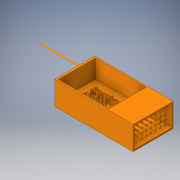
# Autodesk Inventor part: receiver
Saved by Autodesk Inventor 2016 (Build 200138000, 138)
## iProperties
Created: 2015-05-26
Part Number: receiver
Material: Generic
Document SubType Name: Modeling
Designer: Admin
Density: 1 g/cm^3
Appearance: Diamond plate 2 - Dark Gray
Mass: 3.8719 g
Surface Area: 64.7875 cm^2
Volume: 3.8719 cm^3
Author: Admin
Autodesk Inventor part; units mm, degrees
ref_plane "YZ Plane" through (0, 0, 0) normal (1, 0, 0) x (0, 1, 0)
ref_plane "XZ Plane" through (0, 0, 0) normal (0, 1, 0) x (-1, 0, 0)
ref_plane "XY Plane" through (0, 0, 0) normal (0, 0, 1) x (1, 0, 0)
sketch "Sketch1" plane through (0, 0, 0) normal (0, 1, 0) x (-1, 0, 0)
  line L0 (0, 0) -> (43, 0)
  line L1 (43, 0) -> (43, -22)
  line L2 (43, -22) -> (0, -22)
  line L3 (0, -22) -> (0, 0)
  dimension "d0" = 43
  dimension "d1" = 22
  constraints: 8 end point, 2 parallel, 1 horizontal, 1 perpendicular
  measures "d0" distance of L1.end L2.end
  measures "d1" distance of L0.end L1.end
extrude "Extrusion1" add sketch "Sketch1" along normal blind 13
sketch "Sketch2" plane through (0, 0, 0) normal (1, 0, 0) x (0, 0, -1)
  line L0 (0.8065, 0.8735) -> (21.1935, 0.8735)
  line L1 (21.1935, 0.8735) -> (21.1935, 12.1265)
  line L2 (21.1935, 12.1265) -> (0.8065, 12.1265)
  line L3 (0.8065, 12.1265) -> (0.8065, 0.8735)
  line L4 (0.8065, 0.8735) -> (21.1935, 12.1265) construction
  line L5 (21.1935, 0.8735) -> (0.8065, 12.1265) construction
  point P0 (0, 0)
  point P1 (11, 6.5)
  constraints: 12 end point, 2 midpoint, 2 parallel, 1 horizontal, 1 perpendicular
extrude "Extrusion2" cut sketch "Sketch2" against normal blind 13
sketch "Sketch3" plane through (-13, 0, 0) normal (1, 0, 0) x (0, 0, -1)
  circle A0 centre (4.65, 6.5) radius 0.4445
  circle A1 centre (4.65, 9.04) radius 0.4445
  circle A2 centre (4.65, 3.96) radius 0.4445
  line L0 (0.8065, 0.8735) -> (0.8065, 12.1265) projected
  line L1 (21.1935, 12.1265) -> (21.1935, 0.8735) projected
  circle A3 centre (9.73, 6.5) radius 0.4445
  circle A4 centre (9.73, 9.04) radius 0.4445
  circle A5 centre (9.73, 3.96) radius 0.4445
  circle A6 centre (7.19, 9.04) radius 0.4445
  circle A7 centre (7.19, 6.5) radius 0.4445
  circle A8 centre (7.19, 3.96) radius 0.4445
  circle A9 centre (17.35, 6.5) radius 0.4445
  circle A10 centre (17.35, 9.04) radius 0.4445
  circle A11 centre (17.35, 3.96) radius 0.4445
  circle A12 centre (12.27, 9.04) radius 0.4445
  circle A13 centre (12.27, 6.5) radius 0.4445
  circle A14 centre (12.27, 3.96) radius 0.4445
  circle A15 centre (14.81, 9.04) radius 0.4445
  circle A16 centre (14.81, 6.5) radius 0.4445
  circle A17 centre (14.81, 3.96) radius 0.4445
  point P0 (0, 0)
  constraints: 18 centre point
extrude "Extrusion3" add sketch "Sketch3" along normal blind 13
sketch "Sketch4" plane through (0, 13, 0) normal (0, 1, 0) x (1, 0, 0)
  line L0 (-41.9002, 0.8065) -> (-14.0998, 0.8065)
  line L1 (-14.0998, 0.8065) -> (-14.0998, 21.1935)
  line L2 (-14.0998, 21.1935) -> (-41.9002, 21.1935)
  line L3 (-41.9002, 21.1935) -> (-41.9002, 0.8065)
  line L4 (-41.9002, 0.8065) -> (-14.0998, 21.1935) construction
  line L5 (-14.0998, 0.8065) -> (-41.9002, 21.1935) construction
  point P0 (-13, 21.1935)
  point P1 (-13, 0.8065)
  point P2 (-28, 11)
  constraints: 12 end point, 2 midpoint, 2 parallel, 1 horizontal, 1 perpendicular
extrude "Extrusion4" cut sketch "Sketch4" against normal blind 10
sketch "Sketch5" plane through (0, 3, 0) normal (0, 1, 0) x (1, 0, 0)
  line L0 (-36.0677, 15.3871) -> (-11.819, 15.3871) construction
  line L1 (-11.819, 15.3871) -> (-11.819, -1.6232) construction
  line L2 (-11.819, -1.6232) -> (-36.0677, -1.6232) construction
  line L3 (-36.0677, -1.6232) -> (-36.0677, 15.3871) construction
  line L4 (-33.4001, 12.3193) -> (-33.9262, 12.3193)
  line L5 (-33.9262, 12.3193) -> (-34.8895, 13.5321)
  line L6 (-34.8895, 13.5321) -> (-35.3538, 13.5321)
  line L7 (-35.3538, 13.5321) -> (-35.3538, 12.3193)
  line L8 (-35.3538, 12.3193) -> (-35.7589, 12.3193)
  line L9 (-35.7589, 12.3193) -> (-35.7589, 15.3673)
  line L10 (-35.7589, 15.3673) -> (-34.9735, 15.3673)
  spline S0 degree 2 poles (-34.9735, 15.3673) (-34.7116, 15.3673) (-34.3584, 15.3105) (-34.1979, 15.2067) knots 0 0 0 1 2 2 2
  spline S1 degree 2 poles (-34.1979, 15.2067) (-34.0373, 15.103) (-33.8521, 14.7794) (-33.8521, 14.5398) knots 0 0 0 1 2 2 2
  spline S2 degree 2 poles (-33.8521, 14.5398) (-33.8521, 14.2064) (-34.1929, 13.7544) (-34.4844, 13.6457) knots 0 0 0 1 2 2 2
  line L11 (-34.4844, 13.6457) -> (-33.4001, 12.3193)
  spline S3 degree 2 poles (-34.2744, 14.5077) (-34.2744, 14.6411) (-34.3683, 14.8461) (-34.4671, 14.9128) knots 0 0 0 1 2 2 2
  spline S4 degree 2 poles (-34.4671, 14.9128) (-34.5536, 14.9696) (-34.7833, 15.0166) (-34.9512, 15.0166) knots 0 0 0 1 2 2 2
  line L12 (-34.9512, 15.0166) -> (-35.3538, 15.0166)
  line L13 (-35.3538, 15.0166) -> (-35.3538, 13.8705)
  line L14 (-35.3538, 13.8705) -> (-34.9982, 13.8705)
  spline S5 degree 2 poles (-34.9982, 13.8705) (-34.8228, 13.8705) (-34.5437, 13.9322) (-34.4473, 14.0286) knots 0 0 0 1 2 2 2
  spline S6 degree 2 poles (-34.4473, 14.0286) (-34.3584, 14.1125) (-34.2744, 14.3497) (-34.2744, 14.5077) knots 0 0 0 1 2 2 2
  spline S7 degree 2 poles (-32.1947, 12.2674) (-32.743, 12.2674) (-33.3457, 12.8825) (-33.3457, 13.4506) knots 0 0 0 1 2 2 2
  spline S8 degree 2 poles (-33.3457, 13.4506) (-33.3457, 14.0088) (-32.7603, 14.6708) (-32.2886, 14.6708) knots 0 0 0 1 2 2 2
  spline S9 degree 2 poles (-32.2886, 14.6708) (-32.0761, 14.6708) (-31.7476, 14.5473) (-31.6266, 14.4163) knots 0 0 0 1 2 2 2
  spline S10 degree 2 poles (-31.6266, 14.4163) (-31.5031, 14.2854) (-31.3722, 13.9075) (-31.3722, 13.6333) knots 0 0 0 1 2 2 2
  line L15 (-31.3722, 13.6333) -> (-31.3722, 13.4234)
  line L16 (-31.3722, 13.4234) -> (-32.9555, 13.4234)
  spline S11 degree 2 poles (-32.9555, 13.4234) (-32.9555, 13.0257) (-32.5553, 12.6034) (-32.1996, 12.6034) knots 0 0 0 1 2 2 2
  spline S12 degree 2 poles (-32.1996, 12.6034) (-32.0737, 12.6034) (-31.8291, 12.6602) (-31.7303, 12.7046) knots 0 0 0 1 2 2 2
  spline S13 degree 2 poles (-31.7303, 12.7046) (-31.6266, 12.754) (-31.4833, 12.8405) (-31.4364, 12.88) knots 0 0 0 1 2 2 2
  line L17 (-31.4364, 12.88) -> (-31.4142, 12.88)
  line L18 (-31.4142, 12.88) -> (-31.4142, 12.4601)
  spline S14 degree 2 poles (-31.4142, 12.4601) (-31.4809, 12.4329) (-31.6834, 12.3539) (-31.7624, 12.3317) knots 0 0 0 1 2 2 2
  spline S15 degree 2 poles (-31.7624, 12.3317) (-31.8736, 12.2995) (-32.0564, 12.2674) (-32.1947, 12.2674) knots 0 0 0 1 2 2 2
  spline S16 degree 2 poles (-31.7476, 13.7173) (-31.7526, 13.8729) (-31.8168, 14.1002) (-31.8785, 14.1768) knots 0 0 0 1 2 2 2
  spline S17 degree 2 poles (-31.8785, 14.1768) (-31.9452, 14.2632) (-32.1552, 14.3546) (-32.3108, 14.3546) knots 0 0 0 1 2 2 2
  spline S18 degree 2 poles (-32.3108, 14.3546) (-32.4639, 14.3546) (-32.6788, 14.2632) (-32.7677, 14.1743) knots 0 0 0 1 2 2 2
  spline S19 degree 2 poles (-32.7677, 14.1743) (-32.8542, 14.0829) (-32.9431, 13.8631) (-32.9555, 13.7173) knots 0 0 0 1 2 2 2
  line L19 (-32.9555, 13.7173) -> (-31.7476, 13.7173)
  spline S20 degree 2 poles (-30.0729, 12.2674) (-30.3101, 12.2674) (-30.7028, 12.4132) (-30.8436, 12.5614) knots 0 0 0 1 2 2 2
  spline S21 degree 2 poles (-30.8436, 12.5614) (-30.9844, 12.7071) (-31.14, 13.1566) (-31.14, 13.458) knots 0 0 0 1 2 2 2
  spline S22 degree 2 poles (-31.14, 13.458) (-31.14, 13.7593) (-30.9794, 14.199) (-30.8436, 14.3472) knots 0 0 0 1 2 2 2
  spline S23 degree 2 poles (-30.8436, 14.3472) (-30.7077, 14.4979) (-30.3051, 14.6584) (-30.0729, 14.6584) knots 0 0 0 1 2 2 2
  spline S24 degree 2 poles (-30.0729, 14.6584) (-29.8852, 14.6584) (-29.5345, 14.5522) (-29.3986, 14.483) knots 0 0 0 1 2 2 2
  line L20 (-29.3986, 14.483) -> (-29.3986, 14.0508)
  line L21 (-29.3986, 14.0508) -> (-29.4209, 14.0508)
  spline S25 degree 2 poles (-29.4209, 14.0508) (-29.4629, 14.0854) (-29.5913, 14.1743) (-29.6827, 14.2212) knots 0 0 0 1 2 2 2
  spline S26 degree 2 poles (-29.6827, 14.2212) (-29.7642, 14.2607) (-29.9816, 14.3225) (-30.0804, 14.3225) knots 0 0 0 1 2 2 2
  spline S27 degree 2 poles (-30.0804, 14.3225) (-30.3792, 14.3225) (-30.7423, 13.8705) (-30.7423, 13.458) knots 0 0 0 1 2 2 2
  spline S28 degree 2 poles (-30.7423, 13.458) (-30.7423, 13.0554) (-30.3916, 12.6034) (-30.0804, 12.6034) knots 0 0 0 1 2 2 2
  spline S29 degree 2 poles (-30.0804, 12.6034) (-29.8926, 12.6034) (-29.5518, 12.759) (-29.4209, 12.88) knots 0 0 0 1 2 2 2
  line L22 (-29.4209, 12.88) -> (-29.3986, 12.88)
  line L23 (-29.3986, 12.88) -> (-29.3986, 12.4477)
  spline S30 degree 2 poles (-29.3986, 12.4477) (-29.4554, 12.4206) (-29.6283, 12.344) (-29.6975, 12.3267) knots 0 0 0 1 2 2 2
  spline S31 degree 2 poles (-29.6975, 12.3267) (-29.7963, 12.2971) (-29.9519, 12.2674) (-30.0729, 12.2674) knots 0 0 0 1 2 2 2
  spline S32 degree 2 poles (-28.0549, 12.2674) (-28.6033, 12.2674) (-29.206, 12.8825) (-29.206, 13.4506) knots 0 0 0 1 2 2 2
  spline S33 degree 2 poles (-29.206, 13.4506) (-29.206, 14.0088) (-28.6206, 14.6708) (-28.1488, 14.6708) knots 0 0 0 1 2 2 2
  spline S34 degree 2 poles (-28.1488, 14.6708) (-27.9364, 14.6708) (-27.6079, 14.5473) (-27.4868, 14.4163) knots 0 0 0 1 2 2 2
  spline S35 degree 2 poles (-27.4868, 14.4163) (-27.3633, 14.2854) (-27.2324, 13.9075) (-27.2324, 13.6333) knots 0 0 0 1 2 2 2
  line L24 (-27.2324, 13.6333) -> (-27.2324, 13.4234)
  line L25 (-27.2324, 13.4234) -> (-28.8157, 13.4234)
  spline S36 degree 2 poles (-28.8157, 13.4234) (-28.8157, 13.0257) (-28.4156, 12.6034) (-28.0599, 12.6034) knots 0 0 0 1 2 2 2
  spline S37 degree 2 poles (-28.0599, 12.6034) (-27.9339, 12.6034) (-27.6894, 12.6602) (-27.5906, 12.7046) knots 0 0 0 1 2 2 2
  spline S38 degree 2 poles (-27.5906, 12.7046) (-27.4868, 12.754) (-27.3436, 12.8405) (-27.2967, 12.88) knots 0 0 0 1 2 2 2
  line L26 (-27.2967, 12.88) -> (-27.2744, 12.88)
  line L27 (-27.2744, 12.88) -> (-27.2744, 12.4601)
  spline S39 degree 2 poles (-27.2744, 12.4601) (-27.3411, 12.4329) (-27.5437, 12.3539) (-27.6227, 12.3317) knots 0 0 0 1 2 2 2
  spline S40 degree 2 poles (-27.6227, 12.3317) (-27.7338, 12.2995) (-27.9166, 12.2674) (-28.0549, 12.2674) knots 0 0 0 1 2 2 2
  spline S41 degree 2 poles (-27.6079, 13.7173) (-27.6128, 13.8729) (-27.677, 14.1002) (-27.7388, 14.1768) knots 0 0 0 1 2 2 2
  spline S42 degree 2 poles (-27.7388, 14.1768) (-27.8055, 14.2632) (-28.0154, 14.3546) (-28.171, 14.3546) knots 0 0 0 1 2 2 2
  spline S43 degree 2 poles (-28.171, 14.3546) (-28.3242, 14.3546) (-28.5391, 14.2632) (-28.628, 14.1743) knots 0 0 0 1 2 2 2
  spline S44 degree 2 poles (-28.628, 14.1743) (-28.7144, 14.0829) (-28.8034, 13.8631) (-28.8157, 13.7173) knots 0 0 0 1 2 2 2
  line L28 (-28.8157, 13.7173) -> (-27.6079, 13.7173)
  line L29 (-26.4494, 12.3193) -> (-26.8348, 12.3193)
  line L30 (-26.8348, 12.3193) -> (-26.8348, 14.6065)
  line L31 (-26.8348, 14.6065) -> (-26.4494, 14.6065)
  line L32 (-26.4494, 14.6065) -> (-26.4494, 12.3193)
  line L33 (-26.4223, 14.9869) -> (-26.8595, 14.9869)
  line L34 (-26.8595, 14.9869) -> (-26.8595, 15.3871)
  line L35 (-26.8595, 15.3871) -> (-26.4223, 15.3871)
  line L36 (-26.4223, 15.3871) -> (-26.4223, 14.9869)
  line L37 (-24.0881, 14.6065) -> (-24.9501, 12.3193)
  line L38 (-24.9501, 12.3193) -> (-25.2959, 12.3193)
  line L39 (-25.2959, 12.3193) -> (-26.1506, 14.6065)
  line L40 (-26.1506, 14.6065) -> (-25.7331, 14.6065)
  line L41 (-25.7331, 14.6065) -> (-25.1082, 12.8454)
  line L42 (-25.1082, 12.8454) -> (-24.4882, 14.6065)
  line L43 (-24.4882, 14.6065) -> (-24.0881, 14.6065)
  spline S45 degree 2 poles (-22.8037, 12.2674) (-23.352, 12.2674) (-23.9547, 12.8825) (-23.9547, 13.4506) knots 0 0 0 1 2 2 2
  spline S46 degree 2 poles (-23.9547, 13.4506) (-23.9547, 14.0088) (-23.3693, 14.6708) (-22.8976, 14.6708) knots 0 0 0 1 2 2 2
  spline S47 degree 2 poles (-22.8976, 14.6708) (-22.6851, 14.6708) (-22.3566, 14.5473) (-22.2356, 14.4163) knots 0 0 0 1 2 2 2
  spline S48 degree 2 poles (-22.2356, 14.4163) (-22.1121, 14.2854) (-21.9812, 13.9075) (-21.9812, 13.6333) knots 0 0 0 1 2 2 2
  line L44 (-21.9812, 13.6333) -> (-21.9812, 13.4234)
  line L45 (-21.9812, 13.4234) -> (-23.5645, 13.4234)
  spline S49 degree 2 poles (-23.5645, 13.4234) (-23.5645, 13.0257) (-23.1643, 12.6034) (-22.8086, 12.6034) knots 0 0 0 1 2 2 2
  spline S50 degree 2 poles (-22.8086, 12.6034) (-22.6827, 12.6034) (-22.4381, 12.6602) (-22.3393, 12.7046) knots 0 0 0 1 2 2 2
  spline S51 degree 2 poles (-22.3393, 12.7046) (-22.2356, 12.754) (-22.0923, 12.8405) (-22.0454, 12.88) knots 0 0 0 1 2 2 2
  line L46 (-22.0454, 12.88) -> (-22.0232, 12.88)
  line L47 (-22.0232, 12.88) -> (-22.0232, 12.4601)
  spline S52 degree 2 poles (-22.0232, 12.4601) (-22.0899, 12.4329) (-22.2924, 12.3539) (-22.3714, 12.3317) knots 0 0 0 1 2 2 2
  spline S53 degree 2 poles (-22.3714, 12.3317) (-22.4826, 12.2995) (-22.6654, 12.2674) (-22.8037, 12.2674) knots 0 0 0 1 2 2 2
  spline S54 degree 2 poles (-22.3566, 13.7173) (-22.3616, 13.8729) (-22.4258, 14.1002) (-22.4875, 14.1768) knots 0 0 0 1 2 2 2
  spline S55 degree 2 poles (-22.4875, 14.1768) (-22.5542, 14.2632) (-22.7642, 14.3546) (-22.9198, 14.3546) knots 0 0 0 1 2 2 2
  spline S56 degree 2 poles (-22.9198, 14.3546) (-23.0729, 14.3546) (-23.2878, 14.2632) (-23.3767, 14.1743) knots 0 0 0 1 2 2 2
  spline S57 degree 2 poles (-23.3767, 14.1743) (-23.4632, 14.0829) (-23.5521, 13.8631) (-23.5645, 13.7173) knots 0 0 0 1 2 2 2
  line L48 (-23.5645, 13.7173) -> (-22.3566, 13.7173)
  line L49 (-20.3781, 14.194) -> (-20.3979, 14.194)
  spline S58 degree 2 poles (-20.3979, 14.194) (-20.4424, 14.2064) (-20.5387, 14.2113) (-20.6054, 14.2113) knots 0 0 0 1 2 2 2
  spline S59 degree 2 poles (-20.6054, 14.2113) (-20.761, 14.2113) (-21.0673, 14.0755) (-21.2056, 13.9421) knots 0 0 0 1 2 2 2
  line L50 (-21.2056, 13.9421) -> (-21.2056, 12.3193)
  line L51 (-21.2056, 12.3193) -> (-21.5909, 12.3193)
  line L52 (-21.5909, 12.3193) -> (-21.5909, 14.6065)
  line L53 (-21.5909, 14.6065) -> (-21.2056, 14.6065)
  line L54 (-21.2056, 14.6065) -> (-21.2056, 14.2657)
  spline S60 degree 2 poles (-21.2056, 14.2657) (-20.9956, 14.4534) (-20.6819, 14.6065) (-20.5337, 14.6065) knots 0 0 0 1 2 2 2
  spline S61 degree 2 poles (-20.5337, 14.6065) (-20.4745, 14.6065) (-20.4152, 14.6016) (-20.3781, 14.5942) knots 0 0 0 1 2 2 2
  line L55 (-20.3781, 14.5942) -> (-20.3781, 14.194)
  spline S62 degree 2 poles (-34.5684, 7.2465) (-34.8648, 7.2465) (-35.3662, 7.4466) (-35.549, 7.6467) knots 0 0 0 1 2 2 2
  spline S63 degree 2 poles (-35.549, 7.6467) (-35.7318, 7.8443) (-35.9318, 8.4371) (-35.9318, 8.8224) knots 0 0 0 1 2 2 2
  spline S64 degree 2 poles (-35.9318, 8.8224) (-35.9318, 9.2052) (-35.7367, 9.7733) (-35.5514, 9.9833) knots 0 0 0 1 2 2 2
  spline S65 degree 2 poles (-35.5514, 9.9833) (-35.3687, 10.1883) (-34.8697, 10.4032) (-34.561, 10.4032) knots 0 0 0 1 2 2 2
  spline S66 degree 2 poles (-34.561, 10.4032) (-34.4078, 10.4032) (-34.1386, 10.3587) (-34.025, 10.3241) knots 0 0 0 1 2 2 2
  spline S67 degree 2 poles (-34.025, 10.3241) (-33.9262, 10.292) (-33.7212, 10.2006) (-33.6199, 10.1463) knots 0 0 0 1 2 2 2
  line L56 (-33.6199, 10.1463) -> (-33.6199, 9.6572)
  line L57 (-33.6199, 9.6572) -> (-33.652, 9.6572)
  spline S68 degree 2 poles (-33.652, 9.6572) (-33.7063, 9.7066) (-33.8743, 9.845) (-33.9953, 9.9117) knots 0 0 0 1 2 2 2
  spline S69 degree 2 poles (-33.9953, 9.9117) (-34.1114, 9.9759) (-34.3856, 10.0574) (-34.5634, 10.0574) knots 0 0 0 1 2 2 2
  spline S70 degree 2 poles (-34.5634, 10.0574) (-34.7586, 10.0574) (-35.1068, 9.8968) (-35.2378, 9.7437) knots 0 0 0 1 2 2 2
  spline S71 degree 2 poles (-35.2378, 9.7437) (-35.3662, 9.5881) (-35.5095, 9.1163) (-35.5095, 8.8224) knots 0 0 0 1 2 2 2
  spline S72 degree 2 poles (-35.5095, 8.8224) (-35.5095, 8.5087) (-35.3588, 8.0567) (-35.2279, 7.9011) knots 0 0 0 1 2 2 2
  spline S73 degree 2 poles (-35.2279, 7.9011) (-35.0994, 7.7504) (-34.7561, 7.5973) (-34.5634, 7.5973) knots 0 0 0 1 2 2 2
  spline S74 degree 2 poles (-34.5634, 7.5973) (-34.3881, 7.5973) (-34.0892, 7.6837) (-33.9731, 7.7479) knots 0 0 0 1 2 2 2
  spline S75 degree 2 poles (-33.9731, 7.7479) (-33.862, 7.8121) (-33.6965, 7.9455) (-33.6495, 7.9925) knots 0 0 0 1 2 2 2
  line L58 (-33.6495, 7.9925) -> (-33.6199, 7.9925)
  line L59 (-33.6199, 7.9925) -> (-33.6199, 7.5083)
  spline S76 degree 2 poles (-33.6199, 7.5083) (-33.7212, 7.4614) (-33.899, 7.3749) (-34.025, 7.3354) knots 0 0 0 1 2 2 2
  spline S77 degree 2 poles (-34.025, 7.3354) (-34.1584, 7.291) (-34.3856, 7.2465) (-34.5684, 7.2465) knots 0 0 0 1 2 2 2
  line L60 (-32.8789, 7.3008) -> (-33.2642, 7.3008)
  line L61 (-33.2642, 7.3008) -> (-33.2642, 9.5881)
  line L62 (-33.2642, 9.5881) -> (-32.8789, 9.5881)
  line L63 (-32.8789, 9.5881) -> (-32.8789, 7.3008)
  line L64 (-32.8517, 9.9685) -> (-33.2889, 9.9685)
  line L65 (-33.2889, 9.9685) -> (-33.2889, 10.3686)
  line L66 (-33.2889, 10.3686) -> (-32.8517, 10.3686)
  line L67 (-32.8517, 10.3686) -> (-32.8517, 9.9685)
  line L68 (-31.1005, 9.1756) -> (-31.1202, 9.1756)
  spline S78 degree 2 poles (-31.1202, 9.1756) (-31.1647, 9.1879) (-31.261, 9.1929) (-31.3277, 9.1929) knots 0 0 0 1 2 2 2
  spline S79 degree 2 poles (-31.3277, 9.1929) (-31.4833, 9.1929) (-31.7896, 9.057) (-31.9279, 8.9236) knots 0 0 0 1 2 2 2
  line L69 (-31.9279, 8.9236) -> (-31.9279, 7.3008)
  line L70 (-31.9279, 7.3008) -> (-32.3133, 7.3008)
  line L71 (-32.3133, 7.3008) -> (-32.3133, 9.5881)
  line L72 (-32.3133, 9.5881) -> (-31.9279, 9.5881)
  line L73 (-31.9279, 9.5881) -> (-31.9279, 9.2472)
  spline S80 degree 2 poles (-31.9279, 9.2472) (-31.718, 9.4349) (-31.4043, 9.5881) (-31.2561, 9.5881) knots 0 0 0 1 2 2 2
  spline S81 degree 2 poles (-31.2561, 9.5881) (-31.1968, 9.5881) (-31.1375, 9.5831) (-31.1005, 9.5757) knots 0 0 0 1 2 2 2
  line L74 (-31.1005, 9.5757) -> (-31.1005, 9.1756)
  spline S82 degree 2 poles (-29.8926, 7.249) (-30.1298, 7.249) (-30.5225, 7.3947) (-30.6633, 7.5429) knots 0 0 0 1 2 2 2
  spline S83 degree 2 poles (-30.6633, 7.5429) (-30.8041, 7.6886) (-30.9597, 8.1382) (-30.9597, 8.4395) knots 0 0 0 1 2 2 2
  spline S84 degree 2 poles (-30.9597, 8.4395) (-30.9597, 8.7409) (-30.7991, 9.1805) (-30.6633, 9.3287) knots 0 0 0 1 2 2 2
  spline S85 degree 2 poles (-30.6633, 9.3287) (-30.5274, 9.4794) (-30.1248, 9.64) (-29.8926, 9.64) knots 0 0 0 1 2 2 2
  spline S86 degree 2 poles (-29.8926, 9.64) (-29.7049, 9.64) (-29.3542, 9.5337) (-29.2183, 9.4646) knots 0 0 0 1 2 2 2
  line L75 (-29.2183, 9.4646) -> (-29.2183, 9.0323)
  line L76 (-29.2183, 9.0323) -> (-29.2406, 9.0323)
  spline S87 degree 2 poles (-29.2406, 9.0323) (-29.2825, 9.0669) (-29.411, 9.1558) (-29.5024, 9.2028) knots 0 0 0 1 2 2 2
  spline S88 degree 2 poles (-29.5024, 9.2028) (-29.5839, 9.2423) (-29.8012, 9.304) (-29.9, 9.304) knots 0 0 0 1 2 2 2
  spline S89 degree 2 poles (-29.9, 9.304) (-30.1989, 9.304) (-30.562, 8.852) (-30.562, 8.4395) knots 0 0 0 1 2 2 2
  spline S90 degree 2 poles (-30.562, 8.4395) (-30.562, 8.0369) (-30.2113, 7.5849) (-29.9, 7.5849) knots 0 0 0 1 2 2 2
  spline S91 degree 2 poles (-29.9, 7.5849) (-29.7123, 7.5849) (-29.3715, 7.7405) (-29.2406, 7.8615) knots 0 0 0 1 2 2 2
  line L77 (-29.2406, 7.8615) -> (-29.2183, 7.8615)
  line L78 (-29.2183, 7.8615) -> (-29.2183, 7.4293)
  spline S92 degree 2 poles (-29.2183, 7.4293) (-29.2751, 7.4021) (-29.448, 7.3255) (-29.5172, 7.3083) knots 0 0 0 1 2 2 2
  spline S93 degree 2 poles (-29.5172, 7.3083) (-29.616, 7.2786) (-29.7716, 7.249) (-29.8926, 7.249) knots 0 0 0 1 2 2 2
  line L79 (-27.0892, 7.3008) -> (-27.4745, 7.3008)
  line L80 (-27.4745, 7.3008) -> (-27.4745, 7.5528)
  spline S94 degree 2 poles (-27.4745, 7.5528) (-27.6523, 7.3972) (-27.971, 7.2366) (-28.1686, 7.2366) knots 0 0 0 1 2 2 2
  spline S95 degree 2 poles (-28.1686, 7.2366) (-28.3168, 7.2366) (-28.5811, 7.3354) (-28.6774, 7.4416) knots 0 0 0 1 2 2 2
  spline S96 degree 2 poles (-28.6774, 7.4416) (-28.7762, 7.5478) (-28.8849, 7.8714) (-28.8849, 8.1036) knots 0 0 0 1 2 2 2
  line L81 (-28.8849, 8.1036) -> (-28.8849, 9.5881)
  line L82 (-28.8849, 9.5881) -> (-28.4995, 9.5881)
  line L83 (-28.4995, 9.5881) -> (-28.4995, 8.2839)
  spline S97 degree 2 poles (-28.4995, 8.2839) (-28.4995, 8.1011) (-28.4724, 7.8615) (-28.4254, 7.7726) knots 0 0 0 1 2 2 2
  spline S98 degree 2 poles (-28.4254, 7.7726) (-28.3785, 7.6837) (-28.218, 7.6022) (-28.0673, 7.6022) knots 0 0 0 1 2 2 2
  spline S99 degree 2 poles (-28.0673, 7.6022) (-27.9265, 7.6022) (-27.6079, 7.7627) (-27.4745, 7.8788) knots 0 0 0 1 2 2 2
  line L84 (-27.4745, 7.8788) -> (-27.4745, 9.5881)
  line L85 (-27.4745, 9.5881) -> (-27.0892, 9.5881)
  line L86 (-27.0892, 9.5881) -> (-27.0892, 7.3008)
  line L87 (-26.1382, 7.3008) -> (-26.5235, 7.3008)
  line L88 (-26.5235, 7.3008) -> (-26.5235, 9.5881)
  line L89 (-26.5235, 9.5881) -> (-26.1382, 9.5881)
  line L90 (-26.1382, 9.5881) -> (-26.1382, 7.3008)
  line L91 (-26.111, 9.9685) -> (-26.5482, 9.9685)
  line L92 (-26.5482, 9.9685) -> (-26.5482, 10.3686)
  line L93 (-26.5482, 10.3686) -> (-26.111, 10.3686)
  line L94 (-26.111, 10.3686) -> (-26.111, 9.9685)
  spline S100 degree 2 poles (-24.881, 7.2564) (-25.1947, 7.2564) (-25.5479, 7.6145) (-25.5479, 8.0023) knots 0 0 0 1 2 2 2
  line L95 (-25.5479, 8.0023) -> (-25.5479, 9.2695)
  line L96 (-25.5479, 9.2695) -> (-25.8072, 9.2695)
  line L97 (-25.8072, 9.2695) -> (-25.8072, 9.5881)
  line L98 (-25.8072, 9.5881) -> (-25.5479, 9.5881)
  line L99 (-25.5479, 9.5881) -> (-25.5479, 10.2451)
  line L100 (-25.5479, 10.2451) -> (-25.1626, 10.2451)
  line L101 (-25.1626, 10.2451) -> (-25.1626, 9.5881)
  line L102 (-25.1626, 9.5881) -> (-24.4537, 9.5881)
  line L103 (-24.4537, 9.5881) -> (-24.4537, 9.2695)
  line L104 (-24.4537, 9.2695) -> (-25.1626, 9.2695)
  line L105 (-25.1626, 9.2695) -> (-25.1626, 8.1802)
  spline S101 degree 2 poles (-25.1626, 8.1802) (-25.1626, 8.0073) (-25.1502, 7.8171) (-25.1082, 7.7356) knots 0 0 0 1 2 2 2
  spline S102 degree 2 poles (-25.1082, 7.7356) (-25.0736, 7.6639) (-24.918, 7.5923) (-24.7846, 7.5923) knots 0 0 0 1 2 2 2
  spline S103 degree 2 poles (-24.7846, 7.5923) (-24.6908, 7.5923) (-24.5154, 7.6491) (-24.4759, 7.6664) knots 0 0 0 1 2 2 2
  line L106 (-24.4759, 7.6664) -> (-24.4537, 7.6664)
  line L107 (-24.4537, 7.6664) -> (-24.4537, 7.3206)
  spline S104 degree 2 poles (-24.4537, 7.3206) (-24.5623, 7.291) (-24.7846, 7.2564) (-24.881, 7.2564) knots 0 0 0 1 2 2 2
  point P0 (0, 0)
  constraints: 2 other
emboss "Emboss1" sketch "Sketch5" operation add depth 2.54 direction (0, -1, 0)
sketch "Sketch7" plane through (-43, 0, -22) normal (-1, 0, 0) x (0, 0, 1)
  circle A0 centre (2.53, 6.5) radius 0.9525
  point P0 (22, 0)
  dimension "d22" = 1.905
  constraints: 1 centre point
  measures "d22" diameter of A0
extrude "Extrusion6" add sketch "Sketch7" along normal blind 1
sketch "Sketch8" plane through (-44, 6.5, -19.47) normal (-1, 0, 0) x (0, 0, 1)
  circle A0 centre (0, 0) radius 0.3235
  point P0 (19.47, -6.5)
  constraints: 1 centre point
extrude "Extrusion7" add sketch "Sketch8" along normal blind 25.4
body "Solid1"
